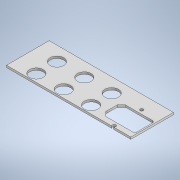
# Autodesk Inventor part: EboxSide
Saved by Autodesk Inventor 2021 (Build 250183000, 183)
## iProperties
Created: 2022-01-03
Part Number: EboxSide
Material: Generic
Document SubType Name: Modeling
Designer: Jorian Brusind
Density: 1 g/cm^3
Appearance: Default
Author: Jorian Brusind
Autodesk Inventor part; units mm, degrees
ref_plane "YZ Plane" through (0, 0, 0) normal (1, 0, 0) x (0, 1, 0)
ref_plane "XZ Plane" through (0, 0, 0) normal (0, 1, 0) x (-1, 0, 0)
ref_plane "XY Plane" through (0, 0, 0) normal (0, 0, 1) x (1, 0, 0)
sketch "Sketch1" plane through (0, 0, 0) normal (0, 1, 0) x (-1, 0, 0)
  line L0 (25.1574, 62.1971) -> (0, 62.1971)
  line L1 (0, 62.1971) -> (0, 0)
  line L2 (0, 0) -> (181.61, 0)
  line L3 (181.61, 0) -> (181.61, 62.1971)
  line L4 (181.61, 62.1971) -> (27.6626, 62.1971)
  line L5 (4.96, 54.5289) -> (44.2742, 54.5289)
  line L6 (44.2742, 54.5289) -> (50.5671, 48.2322)
  line L7 (50.5671, 48.2322) -> (50.5671, 31.808)
  line L8 (50.5671, 31.808) -> (44.2742, 25.5113)
  line L9 (44.2742, 25.5113) -> (4.96, 25.5113)
  ellipse E0 centre (69.3942, 20.866) end of major axis (69.3942, 10.8599) minor radius 10
  ellipse E1 centre (69.3942, 50.8843) end of major axis (69.3942, 40.8782) minor radius 10
  ellipse E2 centre (109.3942, 20.866) end of major axis (109.3942, 10.8599) minor radius 10
  ellipse E3 centre (109.3942, 50.8843) end of major axis (109.3942, 40.8782) minor radius 10
  ellipse E4 centre (149.3942, 50.8843) end of major axis (149.3942, 40.8782) minor radius 10
  ellipse E5 centre (149.3942, 20.866) end of major axis (149.3942, 10.8599) minor radius 10
  ellipse E6 centre (26.41, 60.0323) end of major axis (26.41, 57.5308) minor radius 2.5 (25.1574, 62.1971) -> (27.6626, 62.1971) ccw
  ellipse E7 centre (4.96, 51.5271) end of major axis (4.96, 48.5253) minor radius 3 (4.96, 54.5289) -> (1.96, 51.5271) ccw
  ellipse E8 centre (4.96, 28.5131) end of major axis (4.96, 25.5113) minor radius 3 (1.96, 28.5131) -> (4.96, 25.5113) ccw
  line L10 (1.96, 28.5131) -> (1.96, 51.5271)
  ellipse E9 centre (26.41, 20.0079) end of major axis (26.41, 17.7565) minor radius 2.25
  point P0 (27.6626, 62.1971)
  constraints: 22 end point, 26 other
extrude "Extrusion1" add sketch "Sketch1" along normal blind 3
body "Solid1"
